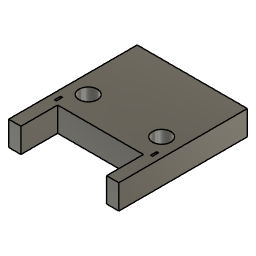
Onderlegplaatje RJ45 female connector v1 (Autodesk Fusion 360 design; units mm, degrees)
Autodesk Fusion 360 part; units mm, degrees
sketch "Sketch1" plane through (0, 0, 0) normal (0, 0, 1) x (1, 0, 0)
  circle A0 centre (2, 10) radius 1.5
  circle A1 centre (14, 10) radius 1.5
  line L0 (-1, 0) -> (17, 0)
  line L1 (17, 0) -> (17, 21)
  line L2 (17, 21) -> (-1, 21)
  line L3 (-1, 21) -> (-1, 0)
  line L4 (0.3, 6.5) -> (0, 6.5)
  line L5 (0, 6.5) -> (0, 7.5)
  line L6 (0, 7.5) -> (0.3, 7.5)
  line L7 (0.3, 7.5) -> (0.3, 6.5)
  line L8 (15.7, 7.5) -> (15.7, 6.5)
  line L9 (16, 7.5) -> (15.7, 7.5)
  line L10 (16, 6.5) -> (16, 7.5)
  line L11 (15.7, 6.5) -> (16, 6.5)
  line L12 (1, 0) -> (1, 6)
  line L13 (1, 6) -> (15, 6)
  line L14 (15, 6) -> (15, 0)
  dimension "d3" = 3
  dimension "d4" = 3
  dimension "d6" = 1
  dimension "d7" = 0.3
  constraint horizontal L0
  constraint vertical L1
  constraint horizontal L2
  constraint vertical L3
  constraint perpendicular L4 L5
  constraint perpendicular L5 L6
  constraint perpendicular L4 L7
  constraint coincident L0 L12.start
  constraint perpendicular L0 L12
  constraint perpendicular L12 L13
  constraint coincident L0 L14.end
  constraint perpendicular L0 L14
  measures "d3" diameter of A0
  measures "d4" diameter of A1
  measures "d6" distance of L4.end L5.end
  measures "d7" distance of L5.end L6.end
extrude "Extrude1" add sketch "Sketch1" along normal blind 4 contours L0 L1 L2 L3 L12 L13 L14
